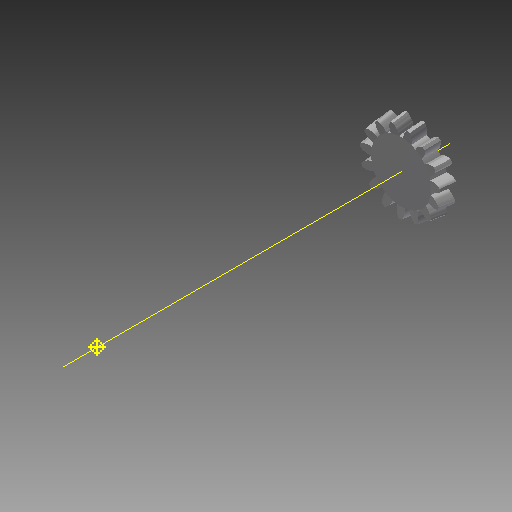
# Autodesk Inventor part: Bevel Gear2
Saved by Autodesk Inventor 2017 (Build 210142000, 142)
## iProperties
Created: 2017-01-10
Part Number: Bevel Gear2
Material: Steel, Mild
Document SubType Name: Modeling
Designer: David Kopala
Categories: <?xml version="1.0" encoding="UTF-16"?> <MemberInstance><Categories><FamilyTemplate><FamilyTemplateParameter ValueType="xs:double" Id="1" ObjectReferenceKey="da_z" ObjectType="kUserParameterObject"/><FamilyTemplateParameter ValueType="xs:double" Id="2" ObjectReferenceKey="da_b" ObjectType="kUserParameterObject"/><FamilyTemplateParameter ValueType="xs:double" Id="3" ObjectReferenceKey="da_beta" ObjectType="kUserParameterObject"/><FamilyTemplateParameter ValueType="xs:double" Id="4" ObjectReferenceKey="da_dae" ObjectType="kUserParameterObject"/><FamilyTemplateParameter ValueType="xs:double" Id="5" ObjectReferenceKey="da_ve" ObjectType="kUserParameterObject"/><FamilyTemplateParameter ValueType="xs:double" Id="6" ObjectReferenceKey="da_omega" ObjectType="kUserParameterObject"/><FamilyTemplateParameter ValueType="xs:string" Id="7" ObjectReferenceKey="EAIAABAAAAAAHwAAAAAAAIAAAAAAAAAA" ObjectType="83914240" SubObjectId="SurfaceGeometry"/></FamilyTemplate><ParamToTemplateMap><ParamToTemplate CategoryParameter="//CategoryParameter[@InternalName='046C89C9-8512-4d59-83FE-43B91F4F132A']" TemplateParameter="1"/><ParamToTemplate CategoryParameter="//CategoryParameter[@InternalName='2552DF32-E462-4b46-AEBF-C6C7768E72AC']" TemplateParameter="2"/><ParamToTemplate CategoryParameter="//CategoryParameter[@InternalName='C9EE641D-15FC-4fae-A226-E94C4372FDD7']" TemplateParameter="3"/><ParamToTemplate><ParamToTemplate CategoryParameter="//CategoryParameter[@InternalName='00B6519A-459B-49c7-AD84-2E56D39A5744']" ConstantValue="-0.000000"/></ParamToTemplate><ParamToTemplate><ParamToTemplate CategoryParameter="//CategoryParameter[@InternalName='04B31F0E-C7A6-4894-AA32-9629BEFACF47']" ConstantValue="1.000000"/></ParamToTemplate><ParamToTemplate><ParamToTemplate CategoryParameter="//CategoryParameter[@InternalName='43CBEC2E-7847-49e7-A936-2F7889FCB2D9']" ConstantValue="0.200000"/></ParamToTemplate><ParamToTemplate><ParamToTemplate CategoryParameter="//CategoryParameter[@InternalName='B1EFC894-105D-4ebd-86BF-FA20ED196853']" ConstantValue="0.300000"/></ParamToTemplate><ParamToTemplate><ParamToTemplate CategoryParameter="//CategoryParameter[@InternalName='51175063-3D10-4879-93E8-6246FE8B403D']" ConstantValue="2061532430.657340"/></ParamToTemplate><ParamToTemplate><ParamToTemplate CategoryParameter="//CategoryParameter[@InternalName='A3A52E27-4454-46a9-B0BD-C932399B70AF']" ConstantValue="0.300000"/></ParamToTemplate><ParamToTemplate CategoryParameter="//CategoryParameter[@InternalName='2A200944-5A8C-41ca-B96E-8520D2E510F1']" TemplateParameter="4"/><ParamToTemplate><ParamToTemplate CategoryParameter="//CategoryParameter[@InternalName='1A637F62-92C8-44bc-B81F-10802510B579']" ConstantValue="4.095423"/></ParamToTemplate><ParamToTemplate CategoryParameter="//CategoryParameter[@InternalName='B52DD4BE-6863-48fb-BF58-89EF6F9EC65C']" TemplateParameter="5"/><ParamToTemplate><ParamToTemplate CategoryParameter="//CategoryParameter[@InternalName='3956BFF2-84D2-457d-93C2-9B0613DEBA67']" ConstantValue="15.472062"/></ParamToTemplate><ParamToTemplate CategoryParameter="//CategoryParameter[@InternalName='739CFA02-461B-4bf8-8049-181FCAD8B28F']" TemplateParameter="6"/><ParamToTemplate><ParamToTemplate CategoryParameter="//CategoryParameter[@InternalName='A27E999F-E2CE-4481-8A2A-EBF499C4C3C5']" ConstantValue="-0.000000"/></ParamToTemplate><ParamToTemplate><ParamToTemplate CategoryParameter="//CategoryParameter[@InternalName='9E1B4470-B2D3-4ff1-B813-535BB4CDF51A']" ConstantValue="3523220.976809"/></ParamToTemplate><ParamToTemplate><ParamToTemplate CategoryParameter="//CategoryParameter[@InternalName='F8452263-BFF6-458c-9FB1-07C4B99E95CD']" ConstantValue="11397033.805607"/></ParamToTemplate><ParamToTemplate><ParamToTemplate CategoryParameter="//CategoryParameter[@InternalName='3E3BB259-FD49-497f-8171-6EBC954A3479']" ConstantValue="2.000000"/></ParamToTemplate><ParamToTemplate CategoryParameter="//CategoryParameter[@InternalName='27C3BAF2-7550-4e4b-AE2C-0DB134B7D9B7']" TemplateParameter="7"/></ParamToTemplateMap><Category DisplayName="Gear" InternalName="DC85795E-93AB-48d5-8EEE-5A27447B64BD" Mnemonic="Gear"><CategoryParameter DisplayName="z" InternalName="046C89C9-8512-4d59-83FE-43B91F4F132A" Mnemonic="z"/><CategoryParameter DisplayName="b" InternalName="2552DF32-E462-4b46-AEBF-C6C7768E72AC" Mnemonic="b"/><CategoryParameter DisplayName="||b|" InternalName="C9EE641D-15FC-4fae-A226-E94C4372FDD7" Mnemonic="beta"/><CategoryParameter DisplayName="x" InternalName="00B6519A-459B-49c7-AD84-2E56D39A5744" Mnemonic="x"/><CategoryParameter DisplayName="a*" InternalName="04B31F0E-C7A6-4894-AA32-9629BEFACF47" Mnemonic="a"/><CategoryParameter DisplayName="c*" InternalName="43CBEC2E-7847-49e7-A936-2F7889FCB2D9" Mnemonic="c"/><CategoryParameter DisplayName="r|.f|*" InternalName="B1EFC894-105D-4ebd-86BF-FA20ED196853" Mnemonic="rf"/><CategoryParameter DisplayName="E" InternalName="51175063-3D10-4879-93E8-6246FE8B403D" Mnemonic="E"/><CategoryParameter DisplayName="||m|" InternalName="A3A52E27-4454-46a9-B0BD-C932399B70AF" Mnemonic="mi"/><Category DisplayName="BevelGear" InternalName="0C98F69A-0C2B-4791-B2FE-7691BB227E77" Mnemonic="BevelGear"><CategoryParameter DisplayName="d|.ae|" InternalName="2A200944-5A8C-41ca-B96E-8520D2E510F1" Mnemonic="dae"/><CategoryParameter DisplayName="d|.ai|" InternalName="1A637F62-92C8-44bc-B81F-10802510B579" Mnemonic="dai"/><CategoryParameter DisplayName="A|.e|" InternalName="B52DD4BE-6863-48fb-BF58-89EF6F9EC65C" Mnemonic="ve"/><CategoryParameter DisplayName="A|.i|" InternalName="3956BFF2-84D2-457d-93C2-9B0613DEBA67" Mnemonic="vi"/><CategoryParameter DisplayName="||S|" InternalName="739CFA02-461B-4bf8-8049-181FCAD8B28F" Mnemonic="omega"/><CategoryParameter DisplayName="x|.t|" InternalName="A27E999F-E2CE-4481-8A2A-EBF499C4C3C5" Mnemonic="xt"/><CategoryParameter DisplayName="||s||.Flim|" InternalName="9E1B4470-B2D3-4ff1-B813-535BB4CDF51A" Mnemonic="sFlim"/><CategoryParameter DisplayName="||s||.Hlim|" InternalName="F8452263-BFF6-458c-9FB1-07C4B99E95CD" Mnemonic="sHlim"/><CategoryParameter DisplayName="type" InternalName="3E3BB259-FD49-497f-8171-6EBC954A3479" Mnemonic="type"/><CategoryParameter DisplayName="PitchDiameter" InternalName="27C3BAF2-7550-4e4b-AE2C-0DB134B7D9B7" Mnemonic="IDS_PITCHDIAM"/></Category></Category></Categories></MemberInstance>
Mass: 60.9118 g
Surface Area: 34.3074 cm^2
Volume: 7.7496 cm^3
Density: 7.86 g/cm^3
Appearance: Steel
CustomPartVersion: 1
Author: David Kopala
Autodesk Inventor part; units mm, degrees
ref_plane "Mesh Plane2" through (0, 0, 0) normal (0.9781476, 0.2079117, 0) x (0, 0, 1)
sketch "Teeth Body Sketch" plane through (0, 0, 0) normal (1, 0, 0) x (0, 1, 0)
  line L0 (0, 0) -> (16.0227, -162.9148) construction
  line L1 (16.0227, -162.9148) -> (21.477, -162.2756)
  line L2 (21.477, -162.2756) -> (0, 0) construction
  line L3 (19.05, -162.56) -> (0, 0) construction
  line L4 (15.2768, -155.33) -> (20.4771, -154.7206)
  line L5 (16.0227, -162.9148) -> (15.2768, -155.33)
  line L6 (21.477, -162.2756) -> (20.4771, -154.7206)
  line L7 (0, -193.977) -> (0, 32.3295) projected
  line L8 (0, -162.56) -> (21.477, -162.56) construction
  dimension "d0" = 38.1
  dimension "d1" = 32.0454
  dimension "d2" = 42.954
  dimension "d3" = 7.62
  dimension "d4" = 162.2756
  constraints: 16 end point, 4 point on line, 3 perpendicular, 2 collinear, 1 horizontal alignment, 1 vertical alignment
  measures "d0" diameter of L3.start L7
  measures "d1" diameter of L0.end L7
  measures "d2" diameter of L1.end L7
  measures "d3" distance between parallel lines of L1 L4
  measures "d4" vertical distance of L1.end L0.start
revolve "Teeth Body" add sketch "Teeth Body Sketch" angle 360 about axis through (0, 0, 0) along (0, 0, 1)
ref_plane "Tooth Plane" through (0, 19.05, -162.56) normal (0, -0.116391, 0.9932035) x (1, 0, 0)
sketch "Start Sketch" plane through (0, 19.05, -162.56) normal (0, -0.116391, 0.9932035) x (1, 0, 0)
  line L0 (0, -23.8473) -> (0, 8.807) projected
  arc A0 (-1.2157, -3.707) -> (-5.7882, 3.3598) centre (-8.4588, -3.381) ccw
  arc A1 (5.7882, 3.3598) -> (1.2157, -3.707) centre (8.4588, -3.381) ccw
  line L1 (-1.2157, -3.707) -> (1.2157, -3.707)
  arc A2 (5.7882, 3.3598) -> (-5.7882, 3.3598) centre (0, -19.1804) ccw
  dimension "d7" = 7.2505
  dimension "d8" = 8.4588
  dimension "d9" = 15.7994
  dimension "d57" = 23.2715
  dimension "d58" = 15.4734
  constraints: 6 point on circle, 3 centre point, 3 symmetric about line, 2 end point, 1 coincident, 1 perpendicular, 1 other
  measures "d7" radius of A0
  measures "d8" horizontal distance of point (0, -19.18) A0.centre
  measures "d9" vertical distance of point (0, -19.18) A0.centre
  measures "d57" radius of A2
  measures "d58" distance from line of A2.centre L1
sketch "End Sketch" plane through (0, 18.1311, -154.7191) normal (0, -0.116391, 0.9932035) x (1, 0, 0)
  line L0 (0, -23.3603) -> (0, 8.4617) projected
  arc A0 (-1.1583, -3.5127) -> (-5.5148, 3.2202) centre (-8.0593, -3.2021) ccw
  arc A1 (5.5148, 3.2202) -> (1.1583, -3.5127) centre (8.0593, -3.2021) ccw
  line L1 (-1.1583, -3.5127) -> (1.1583, -3.5127)
  arc A2 (5.5148, 3.2202) -> (-5.5148, 3.2202) centre (0, -18.2552) ccw
  dimension "d12" = 6.908
  dimension "d15" = 8.0593
  dimension "d16" = 15.0531
  dimension "d59" = 22.1722
  dimension "d60" = 14.7425
  constraints: 6 point on circle, 3 centre point, 3 symmetric about line, 2 end point, 1 coincident, 1 other
  measures "d12" radius of A0
  measures "d15" horizontal distance of A0.centre point (0, -18.255)
  measures "d16" vertical distance of A0.centre point (0, -18.255)
  measures "d59" radius of A2
  measures "d60" distance from line of A2.centre L1
loft "Loft" cut profiles "Start Sketch", "End Sketch"
pattern_circular "Circular Pattern" count 15 over 360 about axis through (0, 0, 0) along (0, 0, 1) of "Loft"
ref_plane "End Plane" through (0, 18.1311, -154.7191) normal (0, -0.116391, 0.9932035) x (1, 0, 0)
sketch3d "3D Sketch Right"
ref_plane "End Plane Right" through (-2.8312, 17.9087, -154.7191) normal (0.0181747, -0.1149633, 0.9932035) x (0.987733, 0.1561522, 0)
sketch "End Sketch Right" plane through (-2.8312, 17.9087, -154.7191) normal (0.0181747, -0.1149633, 0.9932035) x (0.987733, 0.1561522, 0)
  arc A0 (-1.1583, -3.5127) -> (-5.5148, 3.2202) centre (-8.0593, -3.2021) ccw
  line L0 (0, -26.8161) -> (0, 11.9175) projected
  arc A1 (5.5148, 3.2202) -> (1.1583, -3.5127) centre (8.0593, -3.2021) ccw
  line L1 (-1.1583, -3.5127) -> (1.1583, -3.5127)
  arc A2 (5.5148, 3.2202) -> (-5.5148, 3.2202) centre (0, -18.2552) ccw
  dimension "d70" = 8.0593
  dimension "d71" = 15.0531
  dimension "d72" = 6.908
  dimension "d73" = 14.7425
  dimension "d74" = 22.1722
  constraints: 6 point on circle, 3 centre point, 3 symmetric about line, 2 end point, 1 coincident, 1 perpendicular, 1 other
  measures "d70" horizontal distance of A2.centre A0.centre
  measures "d71" vertical distance of point (0, -18.255) A0.centre
  measures "d72" radius of A0
  measures "d73" distance from line of point (0, -18.255) L1
  measures "d74" radius of A2
feature "Loft Right" [suppressed]
pattern_circular "Circular Pattern Right" [suppressed]
sketch3d "3D Sketch Left"
ref_plane "End Plane Left" through (2.82, 17.9087, -154.715) normal (-0.0181031, -0.1149664, 0.9932044) x (0.9878284, -0.1555477, 0)
sketch "End Sketch Left" plane through (2.82, 17.9087, -154.715) normal (-0.0181031, -0.1149664, 0.9932044) x (0.9878284, -0.1555477, 0)
  line L0 (0, -55.8659) -> (0, 21.1697) projected
  arc A0 (-1.1583, -3.5114) -> (-5.5148, 3.2215) centre (-8.0593, -3.2008) ccw
  arc A1 (5.5148, 3.2215) -> (1.1583, -3.5114) centre (8.0593, -3.2008) ccw
  line L1 (-1.1583, -3.5114) -> (1.1583, -3.5114)
  ellipse E0 centre (0, -18.0068) end of major axis (20.4771, -18.0068) minor radius 20.338 projected
  arc A2 (5.5148, 3.2215) -> (-5.5148, 3.2215) centre (0, -18.2539) ccw
  dimension "d56" = 20.338
  dimension "d30" = 6.908
  dimension "d31" = 8.0593
  dimension "d32" = 15.0531
  dimension "d61" = 22.1722
  dimension "d62" = 14.7425
  constraints: 6 point on circle, 3 centre point, 3 symmetric about line, 2 end point, 1 coincident, 2 other
  measures "d30" radius of A0
  measures "d31" horizontal distance of point (0, -18.254) A0.centre
  measures "d32" vertical distance of A0.centre point (0, -18.254)
  measures "d61" radius of A2
  measures "d62" distance from line of point (0, -18.254) L1
feature "Loft Left" [suppressed]
pattern_circular "Circular Pattern Left" [suppressed]
sketch "Body Sketch" plane through (0, 0, 0) normal (1, 0, 0) x (0, 1, 0)
  line L0 (0, -163.1643) -> (0, -152.5465) projected
  line L1 (16.0227, -162.9148) -> (15.2768, -155.33) projected
  line L2 (15.2768, -155.33) -> (0, -155.33)
  line L3 (16.0227, -162.9148) -> (0, -162.9148)
  constraints: 4 end point, 2 perpendicular, 2 point on line
revolve "Fix Body" add sketch "Body Sketch" angle 360 about axis through (0, 0, 0) along (0, 0, 1)
sketch "Sketch6" plane through (0, 0, 0) normal (1, 0, 0) x (0, 1, 0)
  line L0 (19.05, -162.56) -> (0, 0) projected
  line L1 (0, -193.977) -> (0, 32.3295) projected
surface revolve "Pitch Diameter" sketch "Sketch6" angle 360 about axis through (0, 0, 0) along (0, 0, 1) shown no curves L0
sketch "Sketch8" plane through (0, 0, -162.9148) normal (0, 0, -1) x (-1, 0, 0)
  point P0 (0, 0)
  point P1 (0, 0)
  constraints: 1 coincident
equation "\"d0\" = da_de"
equation "\"d1\" = da_dfe"
equation "\"d2\" = da_dae"
equation "\"d3\" = da_b"
equation "\"d4\" = da_ve"
equation "\"d7\" = fd_rr"
equation "\"d8\" = fd_x"
equation "\"d9\" = fd_y"
equation "\"d57\" = 0.5 * fd_dva + 0.3 * da_he"
equation "\"d58\" = 0.5 * fd_dva - 1.12 * da_he"
equation "\"da_teethtype\" = 0"
equation "\"da_b\" = 7.62"
equation "\"da_de\" = 38.1"
equation "\"da_dae\" = 42.95401"
equation "\"da_dfe\" = 32.04543"
equation "\"da_le\" = 163.6724"
equation "\"da_omega\" = 90deg"
equation "\"da_beta\" = 0"
equation "\"da_delta\" = 6.683864deg"
equation "\"da_alpha\" = 20deg"
equation "\"da_he\" = 5.49161"
equation "\"da_ve\" = 162.27559"
equation "\"da_zv\" = 15.102646"
equation "\"fd_loft\" = da_b + 0.05 * da_he"
equation "\"fd_x\" = fd_x1 + fd_x2"
equation "\"fd_y\" = fd_y1 - fd_y2"
equation "\"fd_dd\" = fd_dva - 0.8 * da_he"
equation "\"da_dvw\" = 38.36072"
equation "\"d11\" = fd_loft"
equation "\"da_dm\" = 37.2131"
equation "\"da_x\" = 0"
equation "\"da_m\" = 2.54"
equation "\"d50\" = da_omega"
equation "\"fd_rr\" = 7.250476"
equation "\"fd_dva\" = 43.247949"
equation "\"fd_x1\" = 1.991317"
equation "\"fd_x2\" = 6.467504"
equation "\"fd_y1\" = 19.07671"
equation "\"fd_y2\" = 3.277314"
body "Solid1"
body "Srf1"
